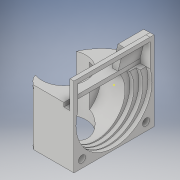
# Autodesk Inventor part: ExtruderCooler
Saved by Autodesk Inventor 2019 (Build 230136000, 136)
## iProperties
Created: 2018-06-27
Part Number: ExtruderCooler
Material: Ogólny
Document SubType Name: Modeling
Designer: Kamil
Density: 1 g/cm^3
Appearance: Domyślna
Author: Kamil
Autodesk Inventor part; units mm, degrees
ref_plane "YZ Plane" through (0, 0, 0) normal (1, 0, 0) x (0, 1, 0)
ref_plane "XZ Plane" through (0, 0, 0) normal (0, 1, 0) x (-1, 0, 0)
ref_plane "XY Plane" through (0, 0, 0) normal (0, 0, 1) x (1, 0, 0)
sketch "Szkic6" plane through (0, 0, 0) normal (0, 1, 0) x (-1, 0, 0)
  line L0 (0, 20) -> (0, -20)
  line L1 (0, 20) -> (40, 20) construction
  arc A0 (24.0003, 15.2468) -> (24.0003, -5.2468) centre (20, 5) ccw
  arc A1 (24.0003, 15.2468) -> (20, 20) centre (15.911, 12.4987) ccw
  line L2 (20, 20) -> (0, 20)
  arc A2 (0, -20) -> (24.0003, -5.2468) centre (1.1842, 4.9719) ccw
  point P0 (0, 0)
  dimension "d22" = 40
  constraints: 6 end point, 6 point on circle, 3 centre point, 2 horizontal, 1 midpoint, 1 perpendicular, 1 vertical
  measures "d22" distance of L0.start L0.end
extrude "Wyciągnięcie proste4" add sketch "Szkic6" along normal blind 26
sketch "Szkic13" plane through (0, 0, 20) normal (1, 0, 0) x (0, 0, -1)
  circle A0 centre (20, 20) radius 19
  point P0 (20, 0)
  dimension "d46" = 38
  constraints: 1 centre point
  measures "d46" diameter of A0
extrude "Wyciągnięcie proste9" cut sketch "Szkic13" against normal blind 2
sketch "Szkic18" plane through (-2, 20, 0) normal (1, 0, 0) x (0, 0, -1)
  circle A0 centre (-1, -1) radius 17.5
  point P0 (0, -20)
  dimension "d52" = 35
  constraints: 1 centre point
  measures "d52" diameter of A0
extrude "Wyciągnięcie proste10" cut sketch "Szkic18" against normal blind 2
sketch "Szkic19" plane through (-4, 19, 1) normal (1, 0, 0) x (0, 0, -1)
  circle A0 centre (-1, -1) radius 16
  point P0 (1, -19)
  dimension "d55" = 32
  constraints: 1 centre point
  measures "d55" diameter of A0
extrude "Wyciągnięcie proste11" cut sketch "Szkic19" against normal blind 2
sketch "Szkic20" plane through (-6, 18, 2) normal (1, 0, 0) x (0, 0, -1)
  circle A0 centre (-1, -1) radius 14.5
  point P0 (2, -18)
  dimension "d58" = 29
  constraints: 1 centre point
  measures "d58" diameter of A0
extrude "Wyciągnięcie proste12" cut sketch "Szkic20" against normal blind 12
sketch "Szkic21" plane through (0, 0, 20) normal (1, 0, 0) x (0, 0, -1)
  circle A0 centre (36, 4) radius 1.75
  circle A1 centre (4, 4) radius 1.75
  point P0 (20, 0)
  dimension "d61" = 3.5
  dimension "d64" = 3.5
  constraints: 2 centre point
  measures "d61" diameter of A0
  measures "d64" diameter of A1
extrude "Wyciągnięcie proste13" cut sketch "Szkic21" against normal blind 10
sketch "Szkic22" plane through (0, 0, 0) normal (0, -1, 0) x (1, 0, 0)
  line L0 (-2.5, -19) -> (-5.5, -19)
  line L1 (-5.5, -19) -> (-5.5, -13)
  line L2 (-5.5, -13) -> (-2.5, -13)
  line L3 (-2.5, -13) -> (-2.5, -19)
  line L4 (-2.5, -19) -> (-5.5, -13) construction
  line L5 (-5.5, -19) -> (-2.5, -13) construction
  line L6 (-2.5, 13) -> (-5.5, 13)
  line L7 (-5.5, 13) -> (-5.5, 19)
  line L8 (-5.5, 19) -> (-2.5, 19)
  line L9 (-2.5, 19) -> (-2.5, 13)
  line L10 (-2.5, 13) -> (-5.5, 19) construction
  line L11 (-5.5, 13) -> (-2.5, 19) construction
  point P0 (0, 0)
  point P1 (-4, -16)
  point P2 (-4, 16)
  dimension "d67" = 3
  dimension "d68" = 6
  dimension "d69" = 3
  dimension "d70" = 6
  constraints: 24 end point, 4 midpoint, 4 parallel, 2 horizontal, 2 perpendicular
  measures "d67" distance of L1.end L2.end
  measures "d68" distance of L0.end L1.end
  measures "d69" distance of L7.end L8.end
  measures "d70" distance of L6.end L7.end
extrude "Wyciągnięcie proste14" cut sketch "Szkic22" against normal blind 7
sketch "Szkic23" plane through (0, 26, 0) normal (0, 1, 0) x (1, 0, 0)
  arc A0 (-24, -15.2639) -> (-21.6936, -18.818) centre (-16.0379, -12.6225) ccw
  arc A1 (-24, -15.247) -> (-23.9955, 5.2487) centre (-20, -5) ccw
  arc A2 (-21.6936, -18.818) -> (-20.0309, -20) centre (-16.0379, -12.6225) ccw
  line L0 (-24, -15.2639) -> (-24, -15.247)
  line L1 (-5, -20) -> (-5, 19.7389)
  line L2 (-5, -20) -> (-20.0309, -20)
  arc A3 (-5, 19.7389) -> (-23.9955, 5.2487) centre (-1.3592, -4.7297) ccw
  point P0 (0, 0)
  point P1 (-24, 5.2384)
  constraints: 10 point on circle, 6 end point, 4 centre point, 1 coincident, 1 horizontal, 1 perpendicular
extrude "Wyciągnięcie proste15" add sketch "Szkic23" along normal blind 2
sketch "Szkic24" plane through (0, 28, 0) normal (0, 1, 0) x (1, 0, 0)
  point P0 (0, 0)
ref_plane "Płaszczyzna konstrukcyjna1" through (-20, 0, -8) normal (0, 0, 1) x (1, 0, 0)
ref_plane "Płaszczyzna konstrukcyjna2" through (-20, 0, -7) normal (0, 0, 1) x (1, 0, 0)
sketch "Szkic25" plane through (-20, 0, -7) normal (0, 0, 1) x (1, 0, 0)
  line L0 (15, 28) -> (12, 28)
  line L1 (12, 28) -> (15, 39.7428)
  line L2 (15, 39.7428) -> (18, 39.7428)
  line L3 (18, 39.7428) -> (15, 28)
  point P0 (20, 0)
  dimension "d78" = 3
  dimension "d79" = 12.12
  dimension "d80" = 3
  constraints: 8 end point, 1 horizontal, 1 parallel
  measures "d78" distance of L0.start L0.end
  measures "d79" distance of L0.end L1.end
  measures "d80" distance of L1.end L2.end
extrude "Wyciągnięcie proste16" add sketch "Szkic25" against normal blind 13
sketch "Szkic26" plane through (-8, 28, -20) normal (0, -1, 0) x (1, 0, 0)
  arc A0 (0, 0.8983) -> (5.5, 0) centre (7.0321, 26.666) ccw
  line L0 (0, 0.8983) -> (0, 0)
  line L1 (0, 0) -> (5.5, 0)
  point P0 (8, 20)
  constraints: 4 end point, 2 point on circle, 1 centre point, 1 perpendicular, 1 vertical
extrude "Wyciągnięcie proste17" cut sketch "Szkic26" against normal blind 12
ref_plane "Płaszczyzna konstrukcyjna3" through (-20, 0, -20) normal (0, 0, 1) x (1, 0, 0)
sketch "Szkic27" plane through (-20, 0, -20) normal (0, 0, 1) x (1, 0, 0)
  line L0 (20, 26) -> (14.9984, 26)
  line L1 (14.9984, 26) -> (14.9984, 28)
  line L2 (14.9984, 28) -> (17.9966, 39.7433)
  line L3 (17.9966, 39.7433) -> (20, 39.7433)
  line L4 (20, 39.7433) -> (20, 26)
  point P0 (20, 0)
  dimension "d85" = 2
  dimension "d86" = 12.12
  constraints: 10 end point, 2 horizontal, 2 perpendicular
  measures "d85" distance of L0.end L1.end
  measures "d86" distance of L1.end L2.end
extrude "Wyciągnięcie proste18" add sketch "Szkic27" along normal blind 2
sketch "Szkic28" plane through (-5, 39.7428, -7) normal (0, 1, 0) x (1, 0, 0)
  line L0 (3, 11) -> (5, 11)
  line L1 (5, 11) -> (5, -27)
  line L2 (5, -27) -> (3, -27)
  line L3 (3, -27) -> (3, 11)
  point P0 (5, -7)
  dimension "d89" = 38
  constraints: 8 end point, 3 perpendicular, 1 horizontal
  measures "d89" distance of L0.end L1.end
extrude "Wyciągnięcie proste19" add sketch "Szkic28" against normal blind 2
sketch "Szkic29" plane through (0, 26, 0) normal (0, 1, 0) x (1, 0, 0)
  line L0 (-2, -20) -> (-2, -18)
  line L1 (-2, -18) -> (0, -18)
  line L2 (0, -18) -> (0, -20)
  line L3 (0, -20) -> (-2, -20)
  point P0 (0, 0)
  dimension "d92" = 2
  dimension "d93" = 2
  dimension "d94" = 2
  constraints: 8 end point, 2 perpendicular, 1 vertical
  measures "d92" distance of L0.start L0.end
  measures "d93" distance of L0.end L1.end
  measures "d94" distance of L1.end L2.end
extrude "Wyciągnięcie proste20" add sketch "Szkic29" along normal blind 12
